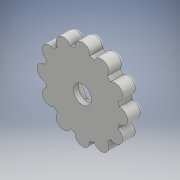
# Autodesk Inventor part: M3-thumbwheel
Saved by Autodesk Inventor 2018 (Build 220112000, 112)
## iProperties
Created: 2017-10-05
Part Number: M3-thumbwheel
Material: Generic
Document SubType Name: Modeling
Designer: leo2a
Density: 1 g/cm^3
Appearance: Default
Author: leo2a
Autodesk Inventor part; units mm, degrees
ref_plane "YZ Plane" through (0, 0, 0) normal (1, 0, 0) x (0, 1, 0)
ref_plane "XZ Plane" through (0, 0, 0) normal (0, 1, 0) x (-1, 0, 0)
ref_plane "XY Plane" through (0, 0, 0) normal (0, 0, 1) x (1, 0, 0)
sketch "Sketch1" plane through (0, 0, 0) normal (0, 1, 0) x (-1, 0, 0)
  circle A0 centre (0, 0) radius 7.5
  circle A1 centre (0, -7.5) radius 1.5
  circle A2 centre (3.75, -6.4952) radius 1.5
  circle A3 centre (6.4952, -3.75) radius 1.5
  circle A4 centre (7.5, 0) radius 1.5
  circle A5 centre (6.4952, 3.75) radius 1.5
  circle A6 centre (3.75, 6.4952) radius 1.5
  circle A7 centre (0, 7.5) radius 1.5
  circle A8 centre (-3.75, 6.4952) radius 1.5
  circle A9 centre (-6.4952, 3.75) radius 1.5
  circle A10 centre (-7.5, 0) radius 1.5
  circle A11 centre (-6.4952, -3.75) radius 1.5
  circle A12 centre (-3.75, -6.4952) radius 1.5
  dimension "d0" = 15
  dimension "d1" = 3
  dimension "d4" = 360
  constraints: 12 centre point, 1 coincident, 1 vertical alignment, 27 other
  measures "d1" diameter of A1
extrude "Extrusion1" add sketch "Sketch1" along normal blind 3
sketch "Sketch2" plane through (0, 3, 0) normal (0, 1, 0) x (1, 0, 0)
  line L0 (0, 0) -> (0, 2.75)
  line L1 (1.5877, 2.75) -> (3.1754, 0)
  line L2 (3.1754, 0) -> (1.5877, -2.75)
  line L3 (1.5877, -2.75) -> (-1.5877, -2.75)
  line L4 (-1.5877, -2.75) -> (-3.1754, 0)
  line L5 (-3.1754, 0) -> (-1.5877, 2.75)
  line L6 (-1.5877, 2.75) -> (1.5877, 2.75)
  dimension "d8" = 2.75
  constraints: 14 end point, 1 coincident, 1 midpoint, 1 vertical, 13 other
  measures "d8" distance of L0.start L0.end
extrude "Extrusion2" cut sketch "Sketch2" against normal blind 2
sketch "Sketch3" plane through (0, 1, 0) normal (0, 1, 0) x (1, 0, 0)
  point P0 (0, 0)
  point P1 (0, 0)
  constraints: 1 coincident
hole "Hole1" at (0, 1, 0) direction (0, -1, 0) diameter 3.6 end through all clearance for "Socket Head Cap Screw" size "M3" standard "Ansi Metric M Profile"
fillet "Fillet1" radius 0.5 24 edges at (7.7942, 3, 4.5) (9, 3, 0) (7.7942, 3, -4.5) (4.5, 3, -7.7942) (0, 3, -9) (-4.5, 3, -7.7942) (-7.7942, 3, -4.5) (-9, 3, 0) (-7.7942, 3, 4.5) (-4.5, 3, 7.7942) (0, 3, 9) (4.5, 3, 7.7942) (5.3033, 3, 5.3033) (7.2444, 3, 1.9411) (7.2444, 3, -1.9411) (5.3033, 3, -5.3033) (1.9411, 3, -7.2444) (-1.9411, 3, -7.2444) (-5.3033, 3, -5.3033) (-7.2444, 3, -1.9411) (-7.2444, 3, 1.9411) (-5.3033, 3, 5.3033) (-1.9411, 3, 7.2444) (1.9411, 3, 7.2444)
fillet "Fillet2" radius 0.5 6 edges at (-2.3816, 3, 1.375) (-2.3816, 3, -1.375) (0, 3, -2.75) (2.3816, 3, -1.375) (2.3816, 3, 1.375) (0, 3, 2.75)
body "Solid1"
